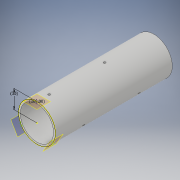
# Autodesk Inventor part: cylinder
Saved by Autodesk Inventor 2017 (Build 210142000, 142)
## iProperties
Part Number: cylinder
Material: Generisch
Document SubType Name: Modeling
Designer: Fabio
Density: 1 g/cm^3
Appearance: Vorgabe
Author: Fabio
Autodesk Inventor part; units mm, degrees
ref_plane "YZ Plane" through (0, 0, 0) normal (1, 0, 0) x (0, 1, 0)
ref_plane "XZ Plane" through (0, 0, 0) normal (0, 1, 0) x (-1, 0, 0)
ref_plane "XY Plane" through (0, 0, 0) normal (0, 0, 1) x (1, 0, 0)
sketch "Skizze1" plane through (0, 0, 0) normal (0, 1, 0) x (-1, 0, 0)
  circle A0 centre (0, 0) radius 27
  circle A1 centre (0, 0) radius 30
  dimension "d0" = 54
  dimension "d10" = 60
  constraints: 2 centre point, 2 coincident
  measures "d0" diameter of A0
  measures "d10" diameter of A1
extrude "Extrusion1" add sketch "Skizze1" along normal blind 190
sketch "Skizze4" plane through (0, 0, 0) normal (0, -1, 0) x (1, 0, 0)
  circle A0 centre (0, 0) radius 30 projected
  point P0 (0, 30)
  point P1 (-25.9808, -15)
  point P2 (25.9808, -15)
  dimension "d11" = 30
  dimension "d14" = 360
  constraints: 1 vertical alignment, 5 other
  measures "d11" distance of point (0, 0) point (0, 30)
ref_plane "Arbeitsebene2" through (0, 0, 30) normal (0, 0, 1) x (1, 0, 0)
ref_plane "Arbeitsebene3" through (25.9808, 0, -15) normal (0.8660254, 0, -0.5) x (0, 1, 0)
ref_plane "Arbeitsebene4" through (-25.9808, 0, -15) normal (-0.8660254, 0, -0.5) x (0, -1, 0)
sketch "Skizze5" plane through (25.9808, 0, -15) normal (0.8660254, 0, -0.5) x (0, 1, 0)
  line L0 (0, 30) -> (0, -30) projected
  line L1 (0, 30) -> (190, 30) projected
  point P0 (0, 0)
  point P1 (50, 0)
  point P2 (140, 0)
  dimension "d16" = 50
  dimension "d17" = 90
  dimension "d18" = 30
  dimension "d19" = 30
  measures "d16" distance from line of point (50, 0) L0
  measures "d17" distance of point (140, 0) point (50, 0)
  measures "d18" distance from line of L1 point (50, 0)
  measures "d19" distance from line of L1 point (140, 0)
sketch "Skizze6" plane through (0, 0, 30) normal (0, 0, 1) x (1, 0, 0)
  line L0 (-30, 0) -> (-30, 190) projected
  line L1 (-30, 0) -> (30, 0) projected
  point P0 (0, 0)
  point P1 (0, 20)
  point P2 (0, 110)
  dimension "d20" = 90
  dimension "d21" = 30
  dimension "d22" = 30
  dimension "d23" = 20
  measures "d20" distance of point (0, 110) point (0, 20)
  measures "d21" distance from line of L0 point (0, 110)
  measures "d22" distance from line of L0 point (0, 20)
  measures "d23" distance from line of L1 point (0, 20)
sketch "Skizze7" plane through (-25.9808, 0, -15) normal (-0.8660254, 0, -0.5) x (0, -1, 0)
  line L0 (0, 30) -> (-190, 30) projected
  point P0 (0, 0)
  point P1 (-80, 0)
  point P2 (-170, 0)
  dimension "d24" = 30
  dimension "d25" = 80
  dimension "d47" = 90
  dimension "d48" = 30
  measures "d24" distance from line of point (-80, 0) L0
  measures "d25" distance of point (0, 0) point (-80, 0)
  measures "d47" distance of point (-80, 0) point (-170, 0)
  measures "d48" distance from line of L0 point (-170, 0)
hole "Bohrung1" at (-25.9808, 80, -15) at (-25.9808, 170, -15) direction (0.8660254, 0, 0.5) diameter 3.3 depth 8 tip angle 118
hole "Bohrung2" at (0, 110, 30) at (0, 20, 30) direction (0, 0, -1) diameter 3.3 depth 8 tip angle 118
hole "Bohrung3" at (25.9808, 50, -15) at (25.9808, 140, -15) direction (-0.8660254, 0, 0.5) diameter 3.3 depth 8 tip angle 118
